Autodesk Fusion 360 part; units mm, degrees
(part 8 of 8)
  spline S237 degree 5 poles (-51.2348, 36.1488) (-51.2355, 36.1491) (-51.2524, 36.1559) (-51.2855, 36.1693) (-51.3349, 36.1892) (-51.4007, 36.2152) (-51.4825, 36.247) (-51.5644, 36.2784) (-51.6466, 36.3093) (-51.7291, 36.3398) (-51.8117, 36.3699) (-51.8946, 36.3996) (-51.9778, 36.4288) (-52.0611, 36.4577) (-52.1447, 36.4861) (-52.2285, 36.5142) (-52.3125, 36.5419) (-52.3966, 36.5692) (-52.481, 36.5962) (-52.5656, 36.6227) (-52.6504, 36.6489) (-52.7353, 36.6747) (-52.8205, 36.7002) (-52.9058, 36.7253) (-52.9913, 36.7501) (-53.077, 36.7745) (-53.1628, 36.7986) (-53.2488, 36.8223) (-53.335, 36.8457) (-53.4214, 36.8688) (-53.5079, 36.8915) (-53.5946, 36.9139) (-53.6814, 36.936) (-53.7684, 36.9577) (-53.8556, 36.9791) (-53.9429, 37.0002) (-54.0304, 37.021) (-54.118, 37.0415) (-54.2057, 37.0616) (-54.2936, 37.0815) (-54.3817, 37.101) (-54.4698, 37.1202) (-54.5582, 37.1391) (-54.6466, 37.1577) (-54.7352, 37.176) (-54.824, 37.1941) (-54.9128, 37.2118) (-55.0018, 37.2292) (-55.091, 37.2463) (-55.1802, 37.2631) (-55.2696, 37.2796) (-55.3591, 37.2958) (-55.4487, 37.3118) (-55.5205, 37.3243) (-55.5745, 37.3336) (-55.6104, 37.3397) (-55.6284, 37.3427) knots 0.270845 0.270845 0.270845 0.270845 0.270845 0.270845 0.271429 0.285714 0.3 0.314286 0.328571 0.342857 0.357143 0.371429 0.385714 0.4 0.414286 0.428571 0.442857 0.457143 0.471429 0.485714 0.5 0.514286 0.528571 0.542857 0.557143 0.571429 0.585714 0.6 0.614286 0.628571 0.642857 0.657143 0.671429 0.685714 0.7 0.714286 0.728571 0.742857 0.757143 0.771429 0.785714 0.8 0.814286 0.828571 0.842857 0.857143 0.871429 0.885714 0.9 0.914286 0.928571 0.942857 0.957143 0.971429 0.985714 1 1 1 1 1 1
  arc A119 (-55.6284, 37.3427) -> (-56.4515, 36.0863) centre (0, 0) ccw
  spline S238 degree 5 poles (-56.4515, 36.0863) (-56.4416, 36.0711) (-56.4216, 36.0405) (-56.3916, 35.9948) (-56.3514, 35.934) (-56.301, 35.8582) (-56.2504, 35.7826) (-56.1995, 35.7072) (-56.1485, 35.6321) (-56.0972, 35.5572) (-56.0457, 35.4826) (-55.994, 35.4082) (-55.942, 35.334) (-55.8899, 35.2601) (-55.8375, 35.1864) (-55.7849, 35.113) (-55.732, 35.0399) (-55.679, 34.9669) (-55.6257, 34.8943) (-55.5721, 34.8219) (-55.5184, 34.7497) (-55.4644, 34.6778) (-55.4102, 34.6062) (-55.3558, 34.5349) (-55.3011, 34.4638) (-55.2462, 34.393) (-55.191, 34.3225) (-55.1356, 34.2522) (-55.08, 34.1823) (-55.0241, 34.1126) (-54.968, 34.0432) (-54.9117, 33.9741) (-54.8551, 33.9053) (-54.7982, 33.8368) (-54.7411, 33.7686) (-54.6837, 33.7007) (-54.6261, 33.6332) (-54.5683, 33.5659) (-54.5101, 33.499) (-54.4517, 33.4324) (-54.3931, 33.3661) (-54.3342, 33.3002) (-54.275, 33.2346) (-54.2155, 33.1693) (-54.1558, 33.1044) (-54.0957, 33.0399) (-54.0354, 32.9757) (-53.9748, 32.912) (-53.9139, 32.8486) (-53.8527, 32.7856) (-53.7913, 32.7229) (-53.7295, 32.6607) (-53.6793, 32.6108) (-53.6414, 32.5734) (-53.6159, 32.5484) (-53.6028, 32.5356) (-53.6023, 32.5351) knots -1 -1 -1 -1 -1 -1 -0.985714 -0.971429 -0.957143 -0.942857 -0.928571 -0.914286 -0.9 -0.885714 -0.871429 -0.857143 -0.842857 -0.828571 -0.814286 -0.8 -0.785714 -0.771429 -0.757143 -0.742857 -0.728571 -0.714286 -0.7 -0.685714 -0.671429 -0.657143 -0.642857 -0.628571 -0.614286 -0.6 -0.585714 -0.571429 -0.557143 -0.542857 -0.528571 -0.514286 -0.5 -0.485714 -0.471429 -0.457143 -0.442857 -0.428571 -0.414286 -0.4 -0.385714 -0.371429 -0.357143 -0.342857 -0.328571 -0.314286 -0.3 -0.285714 -0.271429 -0.270845 -0.270845 -0.270845 -0.270845 -0.270845 -0.270845
  spline S239 degree 3 poles (-53.5708, 32.2888) (-53.5574, 32.3112) (-53.5484, 32.3359) (-53.5405, 32.3873) (-53.5416, 32.4136) (-53.5521, 32.4571) (-53.559, 32.4746) (-53.5775, 32.5072) (-53.5889, 32.5221) (-53.6023, 32.5351) knots 0 0 0 0 0.007813 0.007813 0.015626 0.015626 0.021241 0.021241 0.026855 0.026855 0.026855 0.026855
  arc A120 (-53.5708, 32.2888) -> (-54.254, 31.1273) centre (0, 0) ccw
  spline S240 degree 3 poles (-54.4845, 31.0352) (-54.4596, 31.0278) (-54.4334, 31.0253) (-54.3816, 31.0305) (-54.3564, 31.0381) (-54.3169, 31.0591) (-54.3017, 31.0702) (-54.2748, 31.0963) (-54.2633, 31.1111) (-54.254, 31.1273) knots 0 0 0 0 0.007813 0.007813 0.015626 0.015626 0.021241 0.021241 0.026855 0.026855 0.026855 0.026855
  spline S241 degree 5 poles (-54.4845, 31.0352) (-54.4852, 31.0354) (-54.5027, 31.0406) (-54.5369, 31.0507) (-54.588, 31.0657) (-54.6561, 31.0853) (-54.7405, 31.109) (-54.8251, 31.1323) (-54.9099, 31.1552) (-54.9949, 31.1776) (-55.0801, 31.1996) (-55.1654, 31.2211) (-55.251, 31.2422) (-55.3368, 31.2629) (-55.4227, 31.2831) (-55.5088, 31.303) (-55.595, 31.3224) (-55.6815, 31.3415) (-55.7681, 31.3602) (-55.8548, 31.3784) (-55.9417, 31.3963) (-56.0288, 31.4138) (-56.116, 31.431) (-56.2033, 31.4478) (-56.2908, 31.4642) (-56.3784, 31.4802) (-56.4662, 31.4959) (-56.5541, 31.5112) (-56.6422, 31.5262) (-56.7304, 31.5408) (-56.8187, 31.555) (-56.9071, 31.569) (-56.9957, 31.5826) (-57.0844, 31.5958) (-57.1732, 31.6087) (-57.2621, 31.6213) (-57.3512, 31.6335) (-57.4403, 31.6454) (-57.5296, 31.657) (-57.619, 31.6683) (-57.7086, 31.6792) (-57.7982, 31.6898) (-57.8879, 31.7001) (-57.9778, 31.7101) (-58.0677, 31.7198) (-58.1578, 31.7291) (-58.2479, 31.7382) (-58.3382, 31.7469) (-58.4286, 31.7554) (-58.519, 31.7635) (-58.6096, 31.7713) (-58.7002, 31.7788) (-58.791, 31.786) (-58.8637, 31.7916) (-58.9182, 31.7956) (-58.9546, 31.7982) (-58.9728, 31.7995) knots 0.270845 0.270845 0.270845 0.270845 0.270845 0.270845 0.271429 0.285714 0.3 0.314286 0.328571 0.342857 0.357143 0.371429 0.385714 0.4 0.414286 0.428571 0.442857 0.457143 0.471429 0.485714 0.5 0.514286 0.528571 0.542857 0.557143 0.571429 0.585714 0.6 0.614286 0.628571 0.642857 0.657143 0.671429 0.685714 0.7 0.714286 0.728571 0.742857 0.757143 0.771429 0.785714 0.8 0.814286 0.828571 0.842857 0.857143 0.871429 0.885714 0.9 0.914286 0.928571 0.942857 0.957143 0.971429 0.985714 1 1 1 1 1 1
  arc A121 (-58.9728, 31.7995) -> (-59.6708, 30.4695) centre (0, 0) ccw
  spline S242 degree 5 poles (-59.6708, 30.4695) (-59.6594, 30.4553) (-59.6366, 30.4268) (-59.6023, 30.3842) (-59.5565, 30.3275) (-59.499, 30.2569) (-59.4413, 30.1866) (-59.3834, 30.1165) (-59.3253, 30.0467) (-59.2671, 29.9771) (-59.2086, 29.9078) (-59.15, 29.8387) (-59.0911, 29.7699) (-59.032, 29.7014) (-58.9728, 29.6331) (-58.9133, 29.5651) (-58.8537, 29.4974) (-58.7938, 29.4299) (-58.7338, 29.3627) (-58.6735, 29.2958) (-58.6131, 29.2292) (-58.5524, 29.1629) (-58.4915, 29.0968) (-58.4304, 29.0311) (-58.3692, 28.9656) (-58.3077, 28.9004) (-58.246, 28.8355) (-58.1841, 28.771) (-58.1219, 28.7067) (-58.0596, 28.6427) (-57.9971, 28.5791) (-57.9343, 28.5158) (-57.8713, 28.4527) (-57.8081, 28.3901) (-57.7447, 28.3277) (-57.681, 28.2657) (-57.6172, 28.204) (-57.5531, 28.1426) (-57.4888, 28.0816) (-57.4242, 28.021) (-57.3594, 27.9607) (-57.2944, 27.9007) (-57.2292, 27.8411) (-57.1637, 27.7819) (-57.098, 27.7231) (-57.032, 27.6647) (-56.9658, 27.6066) (-56.8993, 27.549) (-56.8326, 27.4918) (-56.7656, 27.435) (-56.6984, 27.3786) (-56.6309, 27.3226) (-56.5761, 27.2777) (-56.5347, 27.2442) (-56.5069, 27.2217) (-56.4928, 27.2103) (-56.4922, 27.2099) knots -1 -1 -1 -1 -1 -1 -0.985714 -0.971429 -0.957143 -0.942857 -0.928571 -0.914286 -0.9 -0.885714 -0.871429 -0.857143 -0.842857 -0.828571 -0.814286 -0.8 -0.785714 -0.771429 -0.757143 -0.742857 -0.728571 -0.714286 -0.7 -0.685714 -0.671429 -0.657143 -0.642857 -0.628571 -0.614286 -0.6 -0.585714 -0.571429 -0.557143 -0.542857 -0.528571 -0.514286 -0.5 -0.485714 -0.471429 -0.457143 -0.442857 -0.428571 -0.414286 -0.4 -0.385714 -0.371429 -0.357143 -0.342857 -0.328571 -0.314286 -0.3 -0.285714 -0.271429 -0.270845 -0.270845 -0.270845 -0.270845 -0.270845 -0.270845
  spline S243 degree 3 poles (-56.4371, 26.9678) (-56.4258, 26.9913) (-56.4193, 27.0167) (-56.4164, 27.0688) (-56.42, 27.0948) (-56.4346, 27.1371) (-56.4432, 27.1538) (-56.4647, 27.1844) (-56.4776, 27.1982) (-56.4922, 27.2099) knots 0 0 0 0 0.007813 0.007813 0.015626 0.015626 0.021241 0.021241 0.026855 0.026855 0.026855 0.026855
  arc A122 (-56.4371, 26.9678) -> (-57.0049, 25.7458) centre (0, 0) ccw
  spline S244 degree 3 poles (-57.2255, 25.6318) (-57.1999, 25.6268) (-57.1736, 25.6269) (-57.1226, 25.637) (-57.0983, 25.6471) (-57.061, 25.6718) (-57.0469, 25.6843) (-57.0227, 25.7128) (-57.0126, 25.7287) (-57.0049, 25.7458) knots 0 0 0 0 0.007813 0.007813 0.015626 0.015626 0.021241 0.021241 0.026855 0.026855 0.026855 0.026855
  spline S245 degree 5 poles (-57.2255, 25.6318) (-57.2262, 25.6319) (-57.2441, 25.6354) (-57.2791, 25.6422) (-57.3315, 25.6522) (-57.4011, 25.6651) (-57.4874, 25.6806) (-57.5738, 25.6956) (-57.6604, 25.7102) (-57.7472, 25.7243) (-57.8341, 25.7379) (-57.9212, 25.7511) (-58.0084, 25.7638) (-58.0957, 25.7761) (-58.1832, 25.788) (-58.2708, 25.7995) (-58.3586, 25.8105) (-58.4464, 25.8211) (-58.5344, 25.8314) (-58.6225, 25.8412) (-58.7107, 25.8506) (-58.7991, 25.8596) (-58.8875, 25.8683) (-58.9761, 25.8765) (-59.0647, 25.8844) (-59.1535, 25.8919) (-59.2424, 25.8991) (-59.3314, 25.9058) (-59.4205, 25.9122) (-59.5096, 25.9183) (-59.5989, 25.9239) (-59.6883, 25.9293) (-59.7778, 25.9342) (-59.8673, 25.9389) (-59.957, 25.9431) (-60.0467, 25.9471) (-60.1365, 25.9507) (-60.2264, 25.9539) (-60.3164, 25.9568) (-60.4065, 25.9594) (-60.4966, 25.9616) (-60.5869, 25.9636) (-60.6772, 25.9652) (-60.7676, 25.9664) (-60.858, 25.9674) (-60.9486, 25.968) (-61.0392, 25.9683) (-61.1299, 25.9683) (-61.2206, 25.9679) (-61.3114, 25.9673) (-61.4023, 25.9663) (-61.4933, 25.9651) (-61.5843, 25.9635) (-61.6572, 25.962) (-61.7119, 25.9607) (-61.7484, 25.9598) (-61.7666, 25.9593) knots 0.270845 0.270845 0.270845 0.270845 0.270845 0.270845 0.271429 0.285714 0.3 0.314286 0.328571 0.342857 0.357143 0.371429 0.385714 0.4 0.414286 0.428571 0.442857 0.457143 0.471429 0.485714 0.5 0.514286 0.528571 0.542857 0.557143 0.571429 0.585714 0.6 0.614286 0.628571 0.642857 0.657143 0.671429 0.685714 0.7 0.714286 0.728571 0.742857 0.757143 0.771429 0.785714 0.8 0.814286 0.828571 0.842857 0.857143 0.871429 0.885714 0.9 0.914286 0.928571 0.942857 0.957143 0.971429 0.985714 1 1 1 1 1 1
  arc A123 (-61.7666, 25.9593) -> (-62.333, 24.5682) centre (0, 0) ccw
  spline S246 degree 5 poles (-62.333, 24.5682) (-62.3203, 24.5551) (-62.2948, 24.529) (-62.2566, 24.4899) (-62.2055, 24.4379) (-62.1414, 24.3732) (-62.0772, 24.3088) (-62.0129, 24.2446) (-61.9483, 24.1807) (-61.8836, 24.117) (-61.8187, 24.0537) (-61.7537, 23.9906) (-61.6884, 23.9278) (-61.623, 23.8653) (-61.5575, 23.8031) (-61.4917, 23.7411) (-61.4258, 23.6795) (-61.3597, 23.6181) (-61.2935, 23.557) (-61.2271, 23.4962) (-61.1605, 23.4358) (-61.0937, 23.3756) (-61.0267, 23.3157) (-60.9596, 23.2562) (-60.8923, 23.1969) (-60.8248, 23.138) (-60.7571, 23.0794) (-60.6892, 23.0211) (-60.6212, 22.9631) (-60.553, 22.9055) (-60.4846, 22.8481) (-60.416, 22.7912) (-60.3472, 22.7345) (-60.2783, 22.6782) (-60.2091, 22.6223) (-60.1398, 22.5667) (-60.0703, 22.5114) (-60.0006, 22.4566) (-59.9307, 22.402) (-59.8606, 22.3479) (-59.7903, 22.2941) (-59.7198, 22.2408) (-59.6491, 22.1878) (-59.5782, 22.1351) (-59.5071, 22.0829) (-59.4358, 22.0311) (-59.3643, 21.9798) (-59.2925, 21.9288) (-59.2206, 21.8783) (-59.1485, 21.8282) (-59.0761, 21.7786) (-59.0035, 21.7294) (-58.9447, 21.69) (-58.9003, 21.6606) (-58.8704, 21.641) (-58.8552, 21.631) (-58.8546, 21.6306) knots -1 -1 -1 -1 -1 -1 -0.985714 -0.971429 -0.957143 -0.942857 -0.928571 -0.914286 -0.9 -0.885714 -0.871429 -0.857143 -0.842857 -0.828571 -0.814286 -0.8 -0.785714 -0.771429 -0.757143 -0.742857 -0.728571 -0.714286 -0.7 -0.685714 -0.671429 -0.657143 -0.642857 -0.628571 -0.614286 -0.6 -0.585714 -0.571429 -0.557143 -0.542857 -0.528571 -0.514286 -0.5 -0.485714 -0.471429 -0.457143 -0.442857 -0.428571 -0.414286 -0.4 -0.385714 -0.371429 -0.357143 -0.342857 -0.328571 -0.314286 -0.3 -0.285714 -0.271429 -0.270845 -0.270845 -0.270845 -0.270845 -0.270845 -0.270845
  spline S247 degree 3 poles (-58.7764, 21.3949) (-58.7674, 21.4194) (-58.7634, 21.4454) (-58.7655, 21.4974) (-58.7716, 21.523) (-58.7903, 21.5637) (-58.8004, 21.5795) (-58.8248, 21.6079) (-58.839, 21.6203) (-58.8546, 21.6306) knots 0 0 0 0 0.007813 0.007813 0.015626 0.015626 0.021241 0.021241 0.026855 0.026855 0.026855 0.026855
  arc A124 (-58.7764, 21.3949) -> (-59.2236, 20.1238) centre (0, 0) ccw
  spline S248 degree 3 poles (-59.4322, 19.9891) (-59.4062, 19.9866) (-59.3801, 19.9892) (-59.3302, 20.0042) (-59.307, 20.0165) (-59.2723, 20.0448) (-59.2595, 20.0586) (-59.2381, 20.0893) (-59.2296, 20.1061) (-59.2236, 20.1238) knots 0 0 0 0 0.007813 0.007813 0.015626 0.015626 0.021241 0.021241 0.026855 0.026855 0.026855 0.026855
  spline S249 degree 5 poles (-59.4322, 19.9891) (-59.4329, 19.9891) (-59.451, 19.9909) (-59.4866, 19.9943) (-59.5396, 19.9991) (-59.6101, 20.0053) (-59.6975, 20.0124) (-59.785, 20.019) (-59.8726, 20.0251) (-59.9604, 20.0308) (-60.0482, 20.036) (-60.1361, 20.0407) (-60.2242, 20.045) (-60.3123, 20.0488) (-60.4005, 20.0521) (-60.4888, 20.0551) (-60.5772, 20.0576) (-60.6657, 20.0597) (-60.7542, 20.0614) (-60.8429, 20.0627) (-60.9316, 20.0635) (-61.0204, 20.064) (-61.1093, 20.0641) (-61.1982, 20.0637) (-61.2872, 20.063) (-61.3763, 20.0619) (-61.4655, 20.0604) (-61.5547, 20.0586) (-61.644, 20.0564) (-61.7333, 20.0538) (-61.8227, 20.0508) (-61.9122, 20.0475) (-62.0017, 20.0438) (-62.0913, 20.0397) (-62.1809, 20.0353) (-62.2706, 20.0306) (-62.3604, 20.0255) (-62.4502, 20.0201) (-62.54, 20.0143) (-62.6299, 20.0081) (-62.7199, 20.0017) (-62.8099, 19.9949) (-62.8999, 19.9877) (-62.99, 19.9803) (-63.0801, 19.9725) (-63.1703, 19.9644) (-63.2605, 19.9559) (-63.3508, 19.9472) (-63.4411, 19.9381) (-63.5314, 19.9287) (-63.6218, 19.9189) (-63.7122, 19.9089) (-63.8027, 19.8985) (-63.8751, 19.89) (-63.9294, 19.8835) (-63.9656, 19.879) (-63.9837, 19.8768) knots 0.270845 0.270845 0.270845 0.270845 0.270845 0.270845 0.271429 0.285714 0.3 0.314286 0.328571 0.342857 0.357143 0.371429 0.385714 0.4 0.414286 0.428571 0.442857 0.457143 0.471429 0.485714 0.5 0.514286 0.528571 0.542857 0.557143 0.571429 0.585714 0.6 0.614286 0.628571 0.642857 0.657143 0.671429 0.685714 0.7 0.714286 0.728571 0.742857 0.757143 0.771429 0.785714 0.8 0.814286 0.828571 0.842857 0.857143 0.871429 0.885714 0.9 0.914286 0.928571 0.942857 0.957143 0.971429 0.985714 1 1 1 1 1 1
  arc A125 (-63.9837, 19.8768) -> (-64.4132, 18.4375) centre (0, 0) ccw
  spline S250 degree 5 poles (-64.4132, 18.4375) (-64.3993, 18.4257) (-64.3714, 18.4022) (-64.3296, 18.3669) (-64.2737, 18.3201) (-64.2037, 18.2619) (-64.1336, 18.204) (-64.0633, 18.1463) (-63.9929, 18.0889) (-63.9223, 18.0318) (-63.8516, 17.975) (-63.7808, 17.9185) (-63.7098, 17.8623) (-63.6387, 17.8064) (-63.5674, 17.7508) (-63.496, 17.6955) (-63.4245, 17.6405) (-63.3528, 17.5858) (-63.2809, 17.5314) (-63.2089, 17.4773) (-63.1368, 17.4235) (-63.0645, 17.3701) (-62.9921, 17.317) (-62.9195, 17.2642) (-62.8468, 17.2117) (-62.7739, 17.1595) (-62.7009, 17.1077) (-62.6278, 17.0563) (-62.5545, 17.0051) (-62.481, 16.9543) (-62.4074, 16.9039) (-62.3336, 16.8538) (-62.2597, 16.804) (-62.1856, 16.7547) (-62.1114, 16.7057) (-62.037, 16.657) (-61.9625, 16.6087) (-61.8878, 16.5608) (-61.813, 16.5133) (-61.738, 16.4662) (-61.6628, 16.4195) (-61.5875, 16.3731) (-61.512, 16.3272) (-61.4364, 16.2817) (-61.3606, 16.2366) (-61.2846, 16.1919) (-61.2085, 16.1477) (-61.1322, 16.1039) (-61.0557, 16.0605) (-60.9791, 16.0177) (-60.9022, 15.9752) (-60.8252, 15.9333) (-60.7629, 15.8998) (-60.7158, 15.8748) (-60.6843, 15.8581) (-60.6681, 15.8496) (-60.6675, 15.8493) knots -1 -1 -1 -1 -1 -1 -0.985714 -0.971429 -0.957143 -0.942857 -0.928571 -0.914286 -0.9 -0.885714 -0.871429 -0.857143 -0.842857 -0.828571 -0.814286 -0.8 -0.785714 -0.771429 -0.757143 -0.742857 -0.728571 -0.714286 -0.7 -0.685714 -0.671429 -0.657143 -0.642857 -0.628571 -0.614286 -0.6 -0.585714 -0.571429 -0.557143 -0.542857 -0.528571 -0.514286 -0.5 -0.485714 -0.471429 -0.457143 -0.442857 -0.428571 -0.414286 -0.4 -0.385714 -0.371429 -0.357143 -0.342857 -0.328571 -0.314286 -0.3 -0.285714 -0.271429 -0.270845 -0.270845 -0.270845 -0.270845 -0.270845 -0.270845
  spline S251 degree 3 poles (-60.5669, 15.6223) (-60.5604, 15.6475) (-60.5588, 15.6738) (-60.566, 15.7254) (-60.5745, 15.7502) (-60.597, 15.7889) (-60.6086, 15.8037) (-60.6357, 15.8296) (-60.6509, 15.8406) (-60.6675, 15.8493) knots 0 0 0 0 0.007813 0.007813 0.015626 0.015626 0.021241 0.021241 0.026855 0.026855 0.026855 0.026855
  arc A126 (-60.5669, 15.6223) -> (-60.8894, 14.314) centre (0, 0) ccw
  spline S252 degree 3 poles (-61.0839, 14.1597) (-61.0579, 14.1597) (-61.0321, 14.1648) (-60.9839, 14.1846) (-60.962, 14.1992) (-60.9302, 14.2306) (-60.9188, 14.2456) (-60.9005, 14.2782) (-60.8936, 14.2957) (-60.8894, 14.314) knots 0 0 0 0 0.007813 0.007813 0.015626 0.015626 0.021241 0.021241 0.026855 0.026855 0.026855 0.026855
  spline S253 degree 5 poles (-61.0839, 14.1597) (-61.0847, 14.1597) (-61.1029, 14.1597) (-61.1386, 14.1596) (-61.1918, 14.1594) (-61.2626, 14.1587) (-61.3503, 14.1573) (-61.438, 14.1554) (-61.5258, 14.1531) (-61.6137, 14.1503) (-61.7016, 14.1469) (-61.7896, 14.1432) (-61.8776, 14.1389) (-61.9657, 14.1342) (-62.0538, 14.129) (-62.142, 14.1235) (-62.2302, 14.1174) (-62.3185, 14.111) (-62.4068, 14.1041) (-62.4952, 14.0968) (-62.5835, 14.0891) (-62.672, 14.081) (-62.7604, 14.0725) (-62.8489, 14.0636) (-62.9375, 14.0543) (-63.026, 14.0446) (-63.1146, 14.0345) (-63.2032, 14.0241) (-63.2919, 14.0132) (-63.3806, 14.002) (-63.4693, 13.9904) (-63.558, 13.9785) (-63.6468, 13.9662) (-63.7355, 13.9535) (-63.8243, 13.9405) (-63.9132, 13.9271) (-64.002, 13.9134) (-64.0908, 13.8993) (-64.1797, 13.8849) (-64.2686, 13.8701) (-64.3575, 13.855) (-64.4464, 13.8395) (-64.5354, 13.8237) (-64.6243, 13.8076) (-64.7133, 13.7911) (-64.8023, 13.7744) (-64.8912, 13.7572) (-64.9802, 13.7398) (-65.0692, 13.722) (-65.1582, 13.704) (-65.2473, 13.6856) (-65.3363, 13.6668) (-65.4253, 13.6478) (-65.4965, 13.6323) (-65.55, 13.6206) (-65.5856, 13.6127) (-65.6034, 13.6087) knots 0.270845 0.270845 0.270845 0.270845 0.270845 0.270845 0.271429 0.285714 0.3 0.314286 0.328571 0.342857 0.357143 0.371429 0.385714 0.4 0.414286 0.428571 0.442857 0.457143 0.471429 0.485714 0.5 0.514286 0.528571 0.542857 0.557143 0.571429 0.585714 0.6 0.614286 0.628571 0.642857 0.657143 0.671429 0.685714 0.7 0.714286 0.728571 0.742857 0.757143 0.771429 0.785714 0.8 0.814286 0.828571 0.842857 0.857143 0.871429 0.885714 0.9 0.914286 0.928571 0.942857 0.957143 0.971429 0.985714 1 1 1 1 1 1
  arc A127 (-65.6034, 13.6087) -> (-65.892, 12.1347) centre (0, 0) ccw
  spline S254 degree 5 poles (-65.892, 12.1347) (-65.877, 12.1243) (-65.847, 12.1035) (-65.8019, 12.0725) (-65.7418, 12.0313) (-65.6665, 11.9801) (-65.5911, 11.9292) (-65.5156, 11.8786) (-65.44, 11.8283) (-65.3642, 11.7783) (-65.2884, 11.7285) (-65.2124, 11.6791) (-65.1364, 11.63) (-65.0602, 11.5813) (-64.9839, 11.5328) (-64.9075, 11.4846) (-64.8309, 11.4368) (-64.7543, 11.3892) (-64.6775, 11.342) (-64.6007, 11.2952) (-64.5237, 11.2486) (-64.4466, 11.2024) (-64.3694, 11.1565) (-64.292, 11.111) (-64.2146, 11.0657) (-64.137, 11.0209) (-64.0594, 10.9763) (-63.9816, 10.9322) (-63.9037, 10.8884) (-63.8256, 10.8449) (-63.7475, 10.8018) (-63.6693, 10.759) (-63.5909, 10.7167) (-63.5124, 10.6747) (-63.4338, 10.633) (-63.3551, 10.5918) (-63.2762, 10.551) (-63.1973, 10.5105) (-63.1182, 10.4704) (-63.039, 10.4308) (-62.9597, 10.3915) (-62.8802, 10.3526) (-62.8007, 10.3142) (-62.721, 10.2762) (-62.6412, 10.2386) (-62.5613, 10.2015) (-62.4812, 10.1648) (-62.401, 10.1286) (-62.3207, 10.0928) (-62.2403, 10.0576) (-62.1597, 10.0227) (-62.0791, 9.9884) (-62.0137, 9.9611) (-61.9645, 9.9407) (-61.9315, 9.9272) (-61.9146, 9.9203) (-61.914, 9.9201) knots -1 -1 -1 -1 -1 -1 -0.985714 -0.971429 -0.957143 -0.942857 -0.928571 -0.914286 -0.9 -0.885714 -0.871429 -0.857143 -0.842857 -0.828571 -0.814286 -0.8 -0.785714 -0.771429 -0.757143 -0.742857 -0.728571 -0.714286 -0.7 -0.685714 -0.671429 -0.657143 -0.642857 -0.628571 -0.614286 -0.6 -0.585714 -0.571429 -0.557143 -0.542857 -0.528571 -0.514286 -0.5 -0.485714 -0.471429 -0.457143 -0.442857 -0.428571 -0.414286 -0.4 -0.385714 -0.371429 -0.357143 -0.342857 -0.328571 -0.314286 -0.3 -0.285714 -0.271429 -0.270845 -0.270845 -0.270845 -0.270845 -0.270845 -0.270845
  spline S255 degree 3 poles (-61.7919, 9.7038) (-61.7879, 9.7296) (-61.7889, 9.7558) (-61.8009, 9.8065) (-61.8119, 9.8304) (-61.838, 9.8668) (-61.851, 9.8804) (-61.8804, 9.9035) (-61.8966, 9.913) (-61.914, 9.9201) knots 0 0 0 0 0.007813 0.007813 0.015626 0.015626 0.021241 0.021241 0.026855 0.026855 0.026855 0.026855
  arc A128 (-61.7919, 9.7038) -> (-61.9866, 8.3705) centre (0, 0) ccw
  spline S256 degree 3 poles (-62.1654, 8.1982) (-62.1395, 8.2007) (-62.1143, 8.2083) (-62.0682, 8.2326) (-62.0478, 8.2492) (-62.0192, 8.2836) (-62.0093, 8.2996) (-61.9942, 8.3338) (-61.9891, 8.3519) (-61.9866, 8.3705) knots 0 0 0 0 0.007813 0.007813 0.015626 0.015626 0.021241 0.021241 0.026855 0.026855 0.026855 0.026855
  spline S257 degree 5 poles (-62.1654, 8.1982) (-62.1661, 8.1981) (-62.1842, 8.1963) (-62.2198, 8.1928) (-62.2727, 8.1874) (-62.3432, 8.1799) (-62.4303, 8.1701) (-62.5174, 8.1597) (-62.6046, 8.1489) (-62.6918, 8.1376) (-62.779, 8.1258) (-62.8662, 8.1136) (-62.9534, 8.1008) (-63.0406, 8.0877) (-63.1278, 8.074) (-63.215, 8.0599) (-63.3022, 8.0454) (-63.3895, 8.0305) (-63.4767, 8.0151) (-63.5639, 7.9994) (-63.6512, 7.9832) (-63.7384, 7.9666) (-63.8256, 7.9495) (-63.9129, 7.9321) (-64.0001, 7.9143) (-64.0873, 7.8961) (-64.1745, 7.8776) (-64.2617, 7.8586) (-64.3489, 7.8393) (-64.4361, 7.8195) (-64.5233, 7.7995) (-64.6104, 7.779) (-64.6976, 7.7582) (-64.7847, 7.737) (-64.8718, 7.7155) (-64.9589, 7.6936) (-65.046, 7.6713) (-65.1331, 7.6487) (-65.2202, 7.6258) (-65.3072, 7.6025) (-65.3943, 7.5789) (-65.4813, 7.5549) (-65.5683, 7.5306) (-65.6553, 7.506) (-65.7422, 7.481) (-65.8291, 7.4557) (-65.9161, 7.4301) (-66.003, 7.4042) (-66.0898, 7.3779) (-66.1767, 7.3513) (-66.2635, 7.3244) (-66.3503, 7.2972) (-66.4371, 7.2696) (-66.5065, 7.2474) (-66.5585, 7.2305) (-66.5932, 7.2192) (-66.6105, 7.2135) knots 0.270845 0.270845 0.270845 0.270845 0.270845 0.270845 0.271429 0.285714 0.3 0.314286 0.328571 0.342857 0.357143 0.371429 0.385714 0.4 0.414286 0.428571 0.442857 0.457143 0.471429 0.485714 0.5 0.514286 0.528571 0.542857 0.557143 0.571429 0.585714 0.6 0.614286 0.628571 0.642857 0.657143 0.671429 0.685714 0.7 0.714286 0.728571 0.742857 0.757143 0.771429 0.785714 0.8 0.814286 0.828571 0.842857 0.857143 0.871429 0.885714 0.9 0.914286 0.928571 0.942857 0.957143 0.971429 0.985714 1 1 1 1 1 1
  arc A129 (-66.6105, 7.2135) -> (-66.7555, 5.7185) centre (0, 0) ccw
  spline S258 degree 5 poles (-66.7555, 5.7185) (-66.7396, 5.7096) (-66.7077, 5.6919) (-66.6599, 5.6653) (-66.5961, 5.6301) (-66.5162, 5.5864) (-66.4362, 5.543) (-66.3562, 5.5) (-66.2761, 5.4572) (-66.1959, 5.4147) (-66.1156, 5.3725) (-66.0352, 5.3307) (-65.9547, 5.2892) (-65.8742, 5.248) (-65.7936, 5.2071) (-65.7129, 5.1665) (-65.6321, 5.1263) (-65.5512, 5.0864) (-65.4703, 5.0468) (-65.3892, 5.0076) (-65.3081, 4.9687) (-65.2269, 4.9301) (-65.1456, 4.8919) (-65.0643, 4.854) (-64.9828, 4.8165) (-64.9013, 4.7793) (-64.8197, 4.7425) (-64.738, 4.706) (-64.6562, 4.6699) (-64.5744, 4.6342) (-64.4924, 4.5988) (-64.4104, 4.5638) (-64.3283, 4.5292) (-64.2461, 4.495) (-64.1639, 4.4612) (-64.0816, 4.4277) (-63.9991, 4.3947) (-63.9166, 4.362) (-63.8341, 4.3298) (-63.7514, 4.2979) (-63.6687, 4.2665) (-63.5859, 4.2355) (-63.503, 4.2049) (-63.42, 4.1748) (-63.3369, 4.1451) (-63.2538, 4.1158) (-63.1706, 4.0871) (-63.0873, 4.0587) (-63.0039, 4.0309) (-62.9204, 4.0035) (-62.8369, 3.9767) (-62.7533, 3.9503) (-62.6856, 3.9294) (-62.6347, 3.9139) (-62.6005, 3.9036) (-62.583, 3.8984) (-62.5823, 3.8982) knots -1 -1 -1 -1 -1 -1 -0.985714 -0.971429 -0.957143 -0.942857 -0.928571 -0.914286 -0.9 -0.885714 -0.871429 -0.857143 -0.842857 -0.828571 -0.814286 -0.8 -0.785714 -0.771429 -0.757143 -0.742857 -0.728571 -0.714286 -0.7 -0.685714 -0.671429 -0.657143 -0.642857 -0.628571 -0.614286 -0.6 -0.585714 -0.571429 -0.557143 -0.542857 -0.528571 -0.514286 -0.5 -0.485714 -0.471429 -0.457143 -0.442857 -0.428571 -0.414286 -0.4 -0.385714 -0.371429 -0.357143 -0.342857 -0.328571 -0.314286 -0.3 -0.285714 -0.271429 -0.270845 -0.270845 -0.270845 -0.270845 -0.270845 -0.270845
  spline S259 degree 3 poles (-62.44, 3.6948) (-62.4384, 3.7208) (-62.442, 3.7468) (-62.4589, 3.7961) (-62.4721, 3.8188) (-62.5016, 3.8525) (-62.5158, 3.8648) (-62.5473, 3.885) (-62.5644, 3.8928) (-62.5823, 3.8982) knots 0 0 0 0 0.007813 0.007813 0.015626 0.015626 0.021241 0.021241 0.026855 0.026855 0.026855 0.026855
  circle A130 centre (0, 0) radius 10
  circle A131 centre (-30, 0) radius 2
  circle A132 centre (0, -30) radius 2
  circle A133 centre (30, 0) radius 2
  circle A134 centre (0, 30) radius 2
  dimension "d21" = 20
  dimension "d22" = 4
  dimension "d23" = 4
  dimension "d24" = 4
  dimension "d25" = 4
  dimension "d26" = 30
  dimension "d27" = 30
  dimension "d28" = 30
  dimension "d29" = 30
  constraint coincident A0.centre A1.centre
  constraint horizontal A0.centre A131.centre
  constraint vertical A0.centre A132.centre
  constraint horizontal A0.centre A133.centre
  constraint vertical A0.centre A134.centre
  measures "d21" diameter of A130
  measures "d22" diameter of A131
  measures "d23" diameter of A132
  measures "d24" diameter of A133
  measures "d25" diameter of A134
  measures "d26" distance of A0.centre A131.centre
  measures "d27" distance of A0.centre A132.centre
  measures "d28" distance of A0.centre A133.centre
  measures "d29" distance of A0.centre A134.centre
extrude "Extrude3'" cut sketch "Sketch2 (3)" against normal up to surface (5 mm away) contours A130 | A131 | A132 | A133 | A134 bodies 2 in component "Spur Gear (65 teeth)"
component "Spur Gear (15 teeth)" placed x (1, 0, 0) y (0, 1, 0) z (0, 0, 1) at (80, 0, 0)
component "Spur Gear (65 teeth)" placed x (1, 0, 0) y (0, 1, 0) z (0, 0, 1) at (0, 0, 0)
equation "d22 = ScrewDiameter"
equation "d23 = ScrewDiameter"
equation "d24 = ScrewDiameter"
equation "d25 = ScrewDiameter"
equation "ScrewDiameter = 4 mm"
